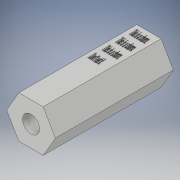
# Autodesk Inventor part: Churro For ARm Gearbox
Saved by Autodesk Inventor 2018 (Build 220112000, 112)
## iProperties
Created: 2019-01-23
Part Number: Churro For ARm Gearbox
Material: Generic
Document SubType Name: Modeling
Designer: Gabriel
Density: 1 g/cm^3
Appearance: Default
Author: Gabriel
Autodesk Inventor part; units mm, degrees
(part 1 of 2)
ref_plane "YZ Plane" through (0, 0, 0) normal (1, 0, 0) x (0, 1, 0)
ref_plane "XZ Plane" through (0, 0, 0) normal (0, 1, 0) x (-1, 0, 0)
ref_plane "XY Plane" through (0, 0, 0) normal (0, 0, 1) x (1, 0, 0)
sketch "Sketch1" plane through (0, 0, 0) normal (0, 0, 1) x (1, 0, 0)
  line L0 (0, 0) -> (0, 6.35) construction
  line L1 (3.6684, 6.35) -> (7.3335, -0.0019)
  line L2 (7.3335, -0.0019) -> (3.6651, -6.3519)
  line L3 (3.6651, -6.3519) -> (-3.6684, -6.35)
  line L4 (-3.6684, -6.35) -> (-7.3335, 0.0019)
  line L5 (-7.3335, 0.0019) -> (-3.6651, 6.3519)
  line L6 (-3.6651, 6.3519) -> (3.6684, 6.35)
  dimension "d0" = 6.35
  constraints: 14 end point, 1 coincident, 1 vertical, 13 other
  measures "d0" distance of L0.start L0.end
extrude "Extrusion1" add sketch "Sketch1" along normal blind 35.56
sketch "Sketch2" plane through (0, 0, 35.56) normal (0, 0, 1) x (1, 0, 0)
  circle A0 centre (0, 0) radius 2.5797
  dimension "d3" = 5.1594
  constraints: 1 centre point, 1 coincident
  measures "d3" diameter of A0
extrude "Extrusion2" cut sketch "Sketch2" against normal blind 38.1
sketch "Sketch3" plane through (-3.6651, 6.3519, 35.56) normal (0.000265, 1, 0) x (1, -0.000265, 0)
  line L0 (1.173, 34.33) -> (52.4364, 34.33) construction
  line L1 (52.4364, 34.33) -> (52.4364, -19.2921) construction
  line L2 (52.4364, -19.2921) -> (1.173, -19.2921) construction
  line L3 (1.173, -19.2921) -> (1.173, 34.33) construction
  line L4 (1.5851, 34.0408) -> (1.4187, 34.0408)
  line L5 (1.4187, 34.0408) -> (1.4187, 31.79)
  line L6 (1.4187, 31.79) -> (1.3533, 31.79)
  line L7 (1.3533, 31.79) -> (1.3533, 34.0408)
  line L8 (1.3533, 34.0408) -> (1.1869, 34.0408)
  line L9 (1.1869, 34.0408) -> (1.1869, 34.33)
  line L10 (1.1869, 34.33) -> (1.5851, 34.33)
  line L11 (1.5851, 34.33) -> (1.5851, 34.0408)
  line L12 (1.9358, 31.79) -> (1.8764, 31.79)
  line L13 (1.8764, 31.79) -> (1.8764, 33.1294)
  spline S0 degree 2 poles (1.8764, 33.1294) (1.8764, 33.2483) (1.8328, 33.4147) (1.8031, 33.4147) knots 0 0 0 1 2 2 2
  spline S1 degree 2 poles (1.8031, 33.4147) (1.7694, 33.4147) (1.706, 33.171) (1.706, 33.0303) knots 0 0 0 1 2 2 2
  line L14 (1.706, 33.0303) -> (1.706, 31.79)
  line L15 (1.706, 31.79) -> (1.6465, 31.79)
  line L16 (1.6465, 31.79) -> (1.6465, 34.33)
  line L17 (1.6465, 34.33) -> (1.706, 34.33)
  line L18 (1.706, 34.33) -> (1.706, 33.4127)
  spline S2 degree 2 poles (1.706, 33.4127) (1.7634, 33.6683) (1.8229, 33.6683) knots 0 0 0 1 1 1
  spline S3 degree 2 poles (1.8229, 33.6683) (1.8684, 33.6683) (1.9358, 33.3929) (1.9358, 33.2086) knots 0 0 0 1 2 2 2
  line L19 (1.9358, 33.2086) -> (1.9358, 31.79)
  line L20 (2.0923, 31.79) -> (2.0329, 31.79)
  line L21 (2.0329, 31.79) -> (2.0329, 33.6188)
  line L22 (2.0329, 33.6188) -> (2.0923, 33.6188)
  line L23 (2.0923, 33.6188) -> (2.0923, 31.79)
  line L24 (2.0923, 33.9675) -> (2.0329, 33.9675)
  line L25 (2.0329, 33.9675) -> (2.0329, 34.33)
  line L26 (2.0329, 34.33) -> (2.0923, 34.33)
  line L27 (2.0923, 34.33) -> (2.0923, 33.9675)
  spline S4 degree 2 poles (2.4609, 32.2913) (2.4609, 32.0238) (2.3776, 31.7128) (2.3142, 31.7128) knots 0 0 0 1 2 2 2
  spline S5 degree 2 poles (2.3142, 31.7128) (2.233, 31.7128) (2.1973, 31.8772) knots 0 0 0 1 1 1
  spline S6 degree 2 poles (2.1973, 31.8772) (2.1676, 32.0159) (2.1656, 32.3289) knots 0 0 0 1 1 1
  line L28 (2.1656, 32.3289) -> (2.2211, 32.3289)
  spline S7 degree 2 poles (2.2211, 32.3289) (2.2211, 32.1447) (2.2508, 32.0436) knots 0 0 0 1 1 1
  spline S8 degree 2 poles (2.2508, 32.0436) (2.2766, 31.9565) (2.3142, 31.9565) knots 0 0 0 1 1 1
  spline S9 degree 2 poles (2.3142, 31.9565) (2.3519, 31.9565) (2.4034, 32.107) (2.4034, 32.2537) knots 0 0 0 1 2 2 2
  spline S10 degree 2 poles (2.4034, 32.2537) (2.4034, 32.4478) (2.3558, 32.5033) knots 0 0 0 1 1 1
  line L29 (2.3558, 32.5033) -> (2.2647, 32.6123)
  spline S11 degree 2 poles (2.2647, 32.6123) (2.2152, 32.6737) (2.1934, 32.8144) knots 0 0 0 1 1 1
  spline S12 degree 2 poles (2.1934, 32.8144) (2.1755, 32.9293) (2.1755, 33.1274) knots 0 0 0 1 1 1
  spline S13 degree 2 poles (2.1755, 33.1274) (2.1755, 33.3751) (2.2528, 33.6703) (2.3162, 33.6703) knots 0 0 0 1 2 2 2
  spline S14 degree 2 poles (2.3162, 33.6703) (2.3776, 33.6703) (2.445, 33.381) (2.447, 33.1056) knots 0 0 0 1 2 2 2
  line L30 (2.447, 33.1056) -> (2.3895, 33.1056)
  spline S15 degree 2 poles (2.3895, 33.1056) (2.3875, 33.3988) (2.3083, 33.3988) knots 0 0 0 1 1 1
  spline S16 degree 2 poles (2.3083, 33.3988) (2.2786, 33.3988) (2.231, 33.2384) (2.231, 33.1175) knots 0 0 0 1 2 2 2
  spline S17 degree 2 poles (2.231, 33.1175) (2.231, 32.9491) (2.2825, 32.8877) knots 0 0 0 1 1 1
  line L31 (2.2825, 32.8877) -> (2.3757, 32.7728)
  spline S18 degree 2 poles (2.3757, 32.7728) (2.4609, 32.6677) (2.4609, 32.2913) knots 0 0 0 1 1 1
  line L32 (2.7897, 31.79) -> (2.7303, 31.79)
  line L33 (2.7303, 31.79) -> (2.7303, 33.6188)
  line L34 (2.7303, 33.6188) -> (2.7897, 33.6188)
  line L35 (2.7897, 33.6188) -> (2.7897, 31.79)
  line L36 (2.7897, 33.9675) -> (2.7303, 33.9675)
  line L37 (2.7303, 33.9675) -> (2.7303, 34.33)
  line L38 (2.7303, 34.33) -> (2.7897, 34.33)
  line L39 (2.7897, 34.33) -> (2.7897, 33.9675)
  spline S19 degree 2 poles (3.1583, 32.2913) (3.1583, 32.0238) (3.075, 31.7128) (3.0116, 31.7128) knots 0 0 0 1 2 2 2
  spline S20 degree 2 poles (3.0116, 31.7128) (2.9304, 31.7128) (2.8948, 31.8772) knots 0 0 0 1 1 1
  spline S21 degree 2 poles (2.8948, 31.8772) (2.865, 32.0159) (2.8631, 32.3289) knots 0 0 0 1 1 1
  line L40 (2.8631, 32.3289) -> (2.9185, 32.3289)
  spline S22 degree 2 poles (2.9185, 32.3289) (2.9185, 32.1447) (2.9482, 32.0436) knots 0 0 0 1 1 1
  spline S23 degree 2 poles (2.9482, 32.0436) (2.974, 31.9565) (3.0116, 31.9565) knots 0 0 0 1 1 1
  spline S24 degree 2 poles (3.0116, 31.9565) (3.0493, 31.9565) (3.1008, 32.107) (3.1008, 32.2537) knots 0 0 0 1 2 2 2
  spline S25 degree 2 poles (3.1008, 32.2537) (3.1008, 32.4478) (3.0533, 32.5033) knots 0 0 0 1 1 1
  line L41 (3.0533, 32.5033) -> (2.9621, 32.6123)
  spline S26 degree 2 poles (2.9621, 32.6123) (2.9126, 32.6737) (2.8908, 32.8144) knots 0 0 0 1 1 1
  spline S27 degree 2 poles (2.8908, 32.8144) (2.873, 32.9293) (2.873, 33.1274) knots 0 0 0 1 1 1
  spline S28 degree 2 poles (2.873, 33.1274) (2.873, 33.3751) (2.9502, 33.6703) (3.0136, 33.6703) knots 0 0 0 1 2 2 2
  spline S29 degree 2 poles (3.0136, 33.6703) (3.075, 33.6703) (3.1424, 33.381) (3.1444, 33.1056) knots 0 0 0 1 2 2 2
  line L42 (3.1444, 33.1056) -> (3.0869, 33.1056)
  spline S30 degree 2 poles (3.0869, 33.1056) (3.085, 33.3988) (3.0057, 33.3988) knots 0 0 0 1 1 1
  spline S31 degree 2 poles (3.0057, 33.3988) (2.976, 33.3988) (2.9284, 33.2384) (2.9284, 33.1175) knots 0 0 0 1 2 2 2
  spline S32 degree 2 poles (2.9284, 33.1175) (2.9284, 32.9491) (2.9799, 32.8877) knots 0 0 0 1 1 1
  line L43 (2.9799, 32.8877) -> (3.0731, 32.7728)
  spline S33 degree 2 poles (3.0731, 32.7728) (3.1583, 32.6677) (3.1583, 32.2913) knots 0 0 0 1 1 1
  spline S34 degree 2 poles (3.7526, 31.7405) (3.7309, 31.7108) (3.7071, 31.7108) knots 0 0 0 1 1 1
  spline S35 degree 2 poles (3.7071, 31.7108) (3.6892, 31.7108) (3.6556, 31.8812) (3.6536, 31.9743) knots 0 0 0 1 2 2 2
  spline S36 degree 2 poles (3.6536, 31.9743) (3.5902, 31.7108) (3.5307, 31.7108) knots 0 0 0 1 1 1
  spline S37 degree 2 poles (3.5307, 31.7108) (3.4753, 31.7108) (3.4099, 31.9961) (3.4099, 32.2477) knots 0 0 0 1 2 2 2
  spline S38 degree 2 poles (3.4099, 32.2477) (3.4099, 32.7212) (3.5228, 32.7985) knots 0 0 0 1 1 1
  line L44 (3.5228, 32.7985) -> (3.6278, 32.8679)
  spline S39 degree 2 poles (3.6278, 32.8679) (3.6516, 32.8857) (3.6516, 33.068) knots 0 0 0 1 1 1
  spline S40 degree 2 poles (3.6516, 33.068) (3.6516, 33.2205) (3.6496, 33.2443) knots 0 0 0 1 1 1
  spline S41 degree 2 poles (3.6496, 33.2443) (3.6437, 33.3176) (3.5902, 33.4087) (3.5565, 33.4087) knots 0 0 0 1 2 2 2
  spline S42 degree 2 poles (3.5565, 33.4087) (3.5228, 33.4087) (3.4872, 33.2522) (3.4812, 33.0719) knots 0 0 0 1 2 2 2
  line L45 (3.4812, 33.0719) -> (3.4277, 33.0719)
  spline S43 degree 2 poles (3.4277, 33.0719) (3.4238, 33.3434) (3.503, 33.6703) (3.5664, 33.6703) knots 0 0 0 1 2 2 2
  spline S44 degree 2 poles (3.5664, 33.6703) (3.6278, 33.6703) (3.713, 33.4543) (3.713, 33.3018) knots 0 0 0 1 2 2 2
  line L46 (3.713, 33.3018) -> (3.713, 32.0654)
  spline S45 degree 2 poles (3.713, 32.0654) (3.713, 32.0278) (3.7269, 31.9664) (3.7368, 31.9584) knots 0 0 0 1 2 2 2
  spline S46 degree 2 poles (3.7368, 31.9584) (3.7427, 31.9545) (3.7526, 31.9584) knots 0 0 0 1 1 1
  line L47 (3.7526, 31.9584) -> (3.7526, 31.7405)
  line L48 (3.6516, 32.3943) -> (3.6516, 32.6777)
  spline S47 degree 2 poles (3.6516, 32.6777) (3.608, 32.6182) (3.5248, 32.5568) knots 0 0 0 1 1 1
  spline S48 degree 2 poles (3.5248, 32.5568) (3.503, 32.535) (3.4713, 32.3606) (3.4713, 32.2517) knots 0 0 0 1 2 2 2
  spline S49 degree 2 poles (3.4713, 32.2517) (3.4713, 32.1269) (3.5089, 31.9584) (3.5367, 31.9584) knots 0 0 0 1 2 2 2
  spline S50 degree 2 poles (3.5367, 31.9584) (3.5842, 31.9584) (3.6516, 32.2239) (3.6516, 32.3943) knots 0 0 0 1 2 2 2
  spline S51 degree 2 poles (4.2935, 32.4201) (4.2856, 32.0377) (4.2381, 31.8554) knots 0 0 0 1 1 1
  spline S52 degree 2 poles (4.2381, 31.8554) (4.2004, 31.7128) (4.143, 31.7128) knots 0 0 0 1 1 1
  spline S53 degree 2 poles (4.143, 31.7128) (4.0697, 31.7128) (3.9825, 32.214) (3.9825, 32.6539) knots 0 0 0 1 2 2 2
  spline S54 degree 2 poles (3.9825, 32.6539) (3.9825, 33.1135) (4.0736, 33.6703) (4.1489, 33.6703) knots 0 0 0 1 2 2 2
  spline S55 degree 2 poles (4.1489, 33.6703) (4.2064, 33.6703) (4.244, 33.5197) knots 0 0 0 1 1 1
  spline S56 degree 2 poles (4.244, 33.5197) (4.2876, 33.3493) (4.2935, 33.0026) knots 0 0 0 1 1 1
  line L49 (4.2935, 33.0026) -> (4.2341, 33.0026)
  spline S57 degree 2 poles (4.2341, 33.0026) (4.2282, 33.3988) (4.1469, 33.3988) knots 0 0 0 1 1 1
  spline S58 degree 2 poles (4.1469, 33.3988) (4.0994, 33.3988) (4.0439, 33.0026) (4.0439, 32.6677) knots 0 0 0 1 2 2 2
  spline S59 degree 2 poles (4.0439, 32.6677) (4.0439, 32.3507) (4.0994, 31.9842) (4.1449, 31.9842) knots 0 0 0 1 2 2 2
  spline S60 degree 2 poles (4.1449, 31.9842) (4.1826, 31.9842) (4.2242, 32.1823) (4.2381, 32.4201) knots 0 0 0 1 2 2 2
  line L50 (4.2381, 32.4201) -> (4.2935, 32.4201)
  line L51 (4.6462, 31.79) -> (4.5868, 31.79)
  line L52 (4.5868, 31.79) -> (4.5868, 33.1294)
  spline S61 degree 2 poles (4.5868, 33.1294) (4.5868, 33.2483) (4.5432, 33.4147) (4.5135, 33.4147) knots 0 0 0 1 2 2 2
  spline S62 degree 2 poles (4.5135, 33.4147) (4.4798, 33.4147) (4.4164, 33.171) (4.4164, 33.0303) knots 0 0 0 1 2 2 2
  line L53 (4.4164, 33.0303) -> (4.4164, 31.79)
  line L54 (4.4164, 31.79) -> (4.3569, 31.79)
  line L55 (4.3569, 31.79) -> (4.3569, 34.33)
  line L56 (4.3569, 34.33) -> (4.4164, 34.33)
  line L57 (4.4164, 34.33) -> (4.4164, 33.4127)
  spline S63 degree 2 poles (4.4164, 33.4127) (4.4738, 33.6683) (4.5333, 33.6683) knots 0 0 0 1 1 1
  spline S64 degree 2 poles (4.5333, 33.6683) (4.5788, 33.6683) (4.6462, 33.3929) (4.6462, 33.2086) knots 0 0 0 1 2 2 2
  line L58 (4.6462, 33.2086) -> (4.6462, 31.79)
  line L59 (5.0345, 31.79) -> (4.9751, 31.79)
  line L60 (4.9751, 31.79) -> (4.9751, 31.9921)
  spline S65 degree 2 poles (4.9751, 31.9921) (4.9533, 31.8376) (4.9295, 31.7782) knots 0 0 0 1 1 1
  spline S66 degree 2 poles (4.9295, 31.7782) (4.9038, 31.7128) (4.8562, 31.7128) knots 0 0 0 1 1 1
  spline S67 degree 2 poles (4.8562, 31.7128) (4.7869, 31.7128) (4.7591, 31.9367) knots 0 0 0 1 1 1
  spline S68 degree 2 poles (4.7591, 31.9367) (4.7433, 32.0575) (4.7433, 32.2081) knots 0 0 0 1 1 1
  line L61 (4.7433, 32.2081) -> (4.7433, 33.6188)
  line L62 (4.7433, 33.6188) -> (4.8027, 33.6188)
  line L63 (4.8027, 33.6188) -> (4.8027, 32.2774)
  spline S69 degree 2 poles (4.8027, 32.2774) (4.8027, 32.1526) (4.8423, 31.9783) (4.8701, 31.9783) knots 0 0 0 1 2 2 2
  spline S70 degree 2 poles (4.8701, 31.9783) (4.9137, 31.9783) (4.9751, 32.2992) (4.9751, 32.5291) knots 0 0 0 1 2 2 2
  line L64 (4.9751, 32.5291) -> (4.9751, 33.6188)
  line L65 (4.9751, 33.6188) -> (5.0345, 33.6188)
  line L66 (5.0345, 33.6188) -> (5.0345, 31.79)
  spline S71 degree 2 poles (5.306, 33.3612) (5.2525, 33.3612) (5.2228, 33.2284) knots 0 0 0 1 1 1
  spline S72 degree 2 poles (5.2228, 33.2284) (5.1891, 33.0818) (5.1891, 32.8144) knots 0 0 0 1 1 1
  line L67 (5.1891, 32.8144) -> (5.1891, 31.79)
  line L68 (5.1891, 31.79) -> (5.1296, 31.79)
  line L69 (5.1296, 31.79) -> (5.1296, 33.6188)
  line L70 (5.1296, 33.6188) -> (5.1891, 33.6188)
  line L71 (5.1891, 33.6188) -> (5.1891, 33.3255)
  spline S73 degree 2 poles (5.1891, 33.3255) (5.2247, 33.6703) (5.2901, 33.6703) knots 0 0 0 1 1 1
  spline S74 degree 2 poles (5.2901, 33.6703) (5.2941, 33.6703) (5.306, 33.6623) knots 0 0 0 1 1 1
  line L72 (5.306, 33.6623) -> (5.306, 33.3612)
  spline S75 degree 2 poles (5.5378, 33.3612) (5.4843, 33.3612) (5.4546, 33.2284) knots 0 0 0 1 1 1
  spline S76 degree 2 poles (5.4546, 33.2284) (5.4209, 33.0818) (5.4209, 32.8144) knots 0 0 0 1 1 1
  line L73 (5.4209, 32.8144) -> (5.4209, 31.79)
  line L74 (5.4209, 31.79) -> (5.3614, 31.79)
  line L75 (5.3614, 31.79) -> (5.3614, 33.6188)
  line L76 (5.3614, 33.6188) -> (5.4209, 33.6188)
  line L77 (5.4209, 33.6188) -> (5.4209, 33.3255)
  spline S77 degree 2 poles (5.4209, 33.3255) (5.4565, 33.6703) (5.5219, 33.6703) knots 0 0 0 1 1 1
  spline S78 degree 2 poles (5.5219, 33.6703) (5.5259, 33.6703) (5.5378, 33.6623) knots 0 0 0 1 1 1
  line L78 (5.5378, 33.6623) -> (5.5378, 33.3612)
  spline S79 degree 2 poles (5.9023, 32.7153) (5.9023, 32.2695) (5.8667, 32.0119) knots 0 0 0 1 1 1
  spline S80 degree 2 poles (5.8667, 32.0119) (5.8231, 31.7128) (5.7379, 31.7128) knots 0 0 0 1 1 1
  spline S81 degree 2 poles (5.7379, 31.7128) (5.6547, 31.7128) (5.6131, 31.9802) knots 0 0 0 1 1 1
  spline S82 degree 2 poles (5.6131, 31.9802) (5.5715, 32.2378) (5.5715, 32.7153) knots 0 0 0 1 1 1
  spline S83 degree 2 poles (5.5715, 32.7153) (5.5715, 33.1611) (5.6567, 33.6703) (5.7379, 33.6703) knots 0 0 0 1 2 2 2
  spline S84 degree 2 poles (5.7379, 33.6703) (5.8171, 33.6703) (5.9023, 33.1611) (5.9023, 32.7153) knots 0 0 0 1 2 2 2
  spline S85 degree 2 poles (5.8409, 32.7153) (5.8409, 33.0264) (5.8092, 33.2106) knots 0 0 0 1 1 1
  spline S86 degree 2 poles (5.8092, 33.2106) (5.7815, 33.377) (5.7379, 33.377) knots 0 0 0 1 1 1
  spline S87 degree 2 poles (5.7379, 33.377) (5.6923, 33.377) (5.6646, 33.2106) knots 0 0 0 1 1 1
  spline S88 degree 2 poles (5.6646, 33.2106) (5.6329, 33.0264) (5.6329, 32.7153) knots 0 0 0 1 1 1
  spline S89 degree 2 poles (5.6329, 32.7153) (5.6329, 32.3923) (5.6903, 32.002) (5.7379, 32.002) knots 0 0 0 1 2 2 2
  spline S90 degree 2 poles (5.7379, 32.002) (5.7835, 32.002) (5.8409, 32.3923) (5.8409, 32.7153) knots 0 0 0 1 2 2 2
  line L79 (6.0648, 31.79) -> (5.9915, 31.79)
  line L80 (5.9915, 31.79) -> (5.9915, 32.1487)
  line L81 (5.9915, 32.1487) -> (6.0648, 32.1487)
  line L82 (6.0648, 32.1487) -> (6.0648, 31.79)
  line L83 (1.5851, 29.9332) -> (1.4187, 29.9332)
  line L84 (1.4187, 29.9332) -> (1.4187, 27.6824)
  line L85 (1.4187, 27.6824) -> (1.3533, 27.6824)
  line L86 (1.3533, 27.6824) -> (1.3533, 29.9332)
  line L87 (1.3533, 29.9332) -> (1.1869, 29.9332)
  line L88 (1.1869, 29.9332) -> (1.1869, 30.2224)
  line L89 (1.1869, 30.2224) -> (1.5851, 30.2224)
  line L90 (1.5851, 30.2224) -> (1.5851, 29.9332)
  line L91 (1.9358, 27.6824) -> (1.8764, 27.6824)
  line L92 (1.8764, 27.6824) -> (1.8764, 29.0218)
  spline S91 degree 2 poles (1.8764, 29.0218) (1.8764, 29.1407) (1.8328, 29.3071) (1.8031, 29.3071) knots 0 0 0 1 2 2 2
  spline S92 degree 2 poles (1.8031, 29.3071) (1.7694, 29.3071) (1.706, 29.0634) (1.706, 28.9227) knots 0 0 0 1 2 2 2
  line L93 (1.706, 28.9227) -> (1.706, 27.6824)
  line L94 (1.706, 27.6824) -> (1.6465, 27.6824)
  line L95 (1.6465, 27.6824) -> (1.6465, 30.2224)
  line L96 (1.6465, 30.2224) -> (1.706, 30.2224)
  line L97 (1.706, 30.2224) -> (1.706, 29.3051)
  spline S93 degree 2 poles (1.706, 29.3051) (1.7634, 29.5607) (1.8229, 29.5607) knots 0 0 0 1 1 1
  spline S94 degree 2 poles (1.8229, 29.5607) (1.8684, 29.5607) (1.9358, 29.2853) (1.9358, 29.101) knots 0 0 0 1 2 2 2
  line L98 (1.9358, 29.101) -> (1.9358, 27.6824)
  line L99 (2.0923, 27.6824) -> (2.0329, 27.6824)
  line L100 (2.0329, 27.6824) -> (2.0329, 29.5112)
  line L101 (2.0329, 29.5112) -> (2.0923, 29.5112)
  line L102 (2.0923, 29.5112) -> (2.0923, 27.6824)
  line L103 (2.0923, 29.8599) -> (2.0329, 29.8599)
  line L104 (2.0329, 29.8599) -> (2.0329, 30.2224)
  line L105 (2.0329, 30.2224) -> (2.0923, 30.2224)
  line L106 (2.0923, 30.2224) -> (2.0923, 29.8599)
  spline S95 degree 2 poles (2.4609, 28.1837) (2.4609, 27.9162) (2.3776, 27.6052) (2.3142, 27.6052) knots 0 0 0 1 2 2 2
  spline S96 degree 2 poles (2.3142, 27.6052) (2.233, 27.6052) (2.1973, 27.7696) knots 0 0 0 1 1 1
  spline S97 degree 2 poles (2.1973, 27.7696) (2.1676, 27.9083) (2.1656, 28.2213) knots 0 0 0 1 1 1
  line L107 (2.1656, 28.2213) -> (2.2211, 28.2213)
  spline S98 degree 2 poles (2.2211, 28.2213) (2.2211, 28.0371) (2.2508, 27.936) knots 0 0 0 1 1 1
  spline S99 degree 2 poles (2.2508, 27.936) (2.2766, 27.8489) (2.3142, 27.8489) knots 0 0 0 1 1 1
  spline S100 degree 2 poles (2.3142, 27.8489) (2.3519, 27.8489) (2.4034, 27.9994) (2.4034, 28.1461) knots 0 0 0 1 2 2 2
  spline S101 degree 2 poles (2.4034, 28.1461) (2.4034, 28.3402) (2.3558, 28.3957) knots 0 0 0 1 1 1
  line L108 (2.3558, 28.3957) -> (2.2647, 28.5047)
  spline S102 degree 2 poles (2.2647, 28.5047) (2.2152, 28.5661) (2.1934, 28.7068) knots 0 0 0 1 1 1
  spline S103 degree 2 poles (2.1934, 28.7068) (2.1755, 28.8217) (2.1755, 29.0198) knots 0 0 0 1 1 1
  spline S104 degree 2 poles (2.1755, 29.0198) (2.1755, 29.2675) (2.2528, 29.5627) (2.3162, 29.5627) knots 0 0 0 1 2 2 2
  spline S105 degree 2 poles (2.3162, 29.5627) (2.3776, 29.5627) (2.445, 29.2734) (2.447, 28.998) knots 0 0 0 1 2 2 2
  line L109 (2.447, 28.998) -> (2.3895, 28.998)
  spline S106 degree 2 poles (2.3895, 28.998) (2.3875, 29.2912) (2.3083, 29.2912) knots 0 0 0 1 1 1
  spline S107 degree 2 poles (2.3083, 29.2912) (2.2786, 29.2912) (2.231, 29.1308) (2.231, 29.0099) knots 0 0 0 1 2 2 2
  spline S108 degree 2 poles (2.231, 29.0099) (2.231, 28.8415) (2.2825, 28.7801) knots 0 0 0 1 1 1
  line L110 (2.2825, 28.7801) -> (2.3757, 28.6652)
  spline S109 degree 2 poles (2.3757, 28.6652) (2.4609, 28.5601) (2.4609, 28.1837) knots 0 0 0 1 1 1
  line L111 (2.7897, 27.6824) -> (2.7303, 27.6824)
  line L112 (2.7303, 27.6824) -> (2.7303, 29.5112)
  line L113 (2.7303, 29.5112) -> (2.7897, 29.5112)
  line L114 (2.7897, 29.5112) -> (2.7897, 27.6824)
  line L115 (2.7897, 29.8599) -> (2.7303, 29.8599)
  line L116 (2.7303, 29.8599) -> (2.7303, 30.2224)
  line L117 (2.7303, 30.2224) -> (2.7897, 30.2224)
  line L118 (2.7897, 30.2224) -> (2.7897, 29.8599)
  spline S110 degree 2 poles (3.1583, 28.1837) (3.1583, 27.9162) (3.075, 27.6052) (3.0116, 27.6052) knots 0 0 0 1 2 2 2
  spline S111 degree 2 poles (3.0116, 27.6052) (2.9304, 27.6052) (2.8948, 27.7696) knots 0 0 0 1 1 1
  spline S112 degree 2 poles (2.8948, 27.7696) (2.865, 27.9083) (2.8631, 28.2213) knots 0 0 0 1 1 1
  line L119 (2.8631, 28.2213) -> (2.9185, 28.2213)
  spline S113 degree 2 poles (2.9185, 28.2213) (2.9185, 28.0371) (2.9482, 27.936) knots 0 0 0 1 1 1
  spline S114 degree 2 poles (2.9482, 27.936) (2.974, 27.8489) (3.0116, 27.8489) knots 0 0 0 1 1 1
  spline S115 degree 2 poles (3.0116, 27.8489) (3.0493, 27.8489) (3.1008, 27.9994) (3.1008, 28.1461) knots 0 0 0 1 2 2 2
  spline S116 degree 2 poles (3.1008, 28.1461) (3.1008, 28.3402) (3.0533, 28.3957) knots 0 0 0 1 1 1
  line L120 (3.0533, 28.3957) -> (2.9621, 28.5047)
  spline S117 degree 2 poles (2.9621, 28.5047) (2.9126, 28.5661) (2.8908, 28.7068) knots 0 0 0 1 1 1
  spline S118 degree 2 poles (2.8908, 28.7068) (2.873, 28.8217) (2.873, 29.0198) knots 0 0 0 1 1 1
  spline S119 degree 2 poles (2.873, 29.0198) (2.873, 29.2675) (2.9502, 29.5627) (3.0136, 29.5627) knots 0 0 0 1 2 2 2
  spline S120 degree 2 poles (3.0136, 29.5627) (3.075, 29.5627) (3.1424, 29.2734) (3.1444, 28.998) knots 0 0 0 1 2 2 2
  line L121 (3.1444, 28.998) -> (3.0869, 28.998)
  spline S121 degree 2 poles (3.0869, 28.998) (3.085, 29.2912) (3.0057, 29.2912) knots 0 0 0 1 1 1
  spline S122 degree 2 poles (3.0057, 29.2912) (2.976, 29.2912) (2.9284, 29.1308) (2.9284, 29.0099) knots 0 0 0 1 2 2 2
  spline S123 degree 2 poles (2.9284, 29.0099) (2.9284, 28.8415) (2.9799, 28.7801) knots 0 0 0 1 1 1
  line L122 (2.9799, 28.7801) -> (3.0731, 28.6652)
  spline S124 degree 2 poles (3.0731, 28.6652) (3.1583, 28.5601) (3.1583, 28.1837) knots 0 0 0 1 1 1
  spline S125 degree 2 poles (3.7526, 27.6329) (3.7309, 27.6032) (3.7071, 27.6032) knots 0 0 0 1 1 1
  spline S126 degree 2 poles (3.7071, 27.6032) (3.6892, 27.6032) (3.6556, 27.7736) (3.6536, 27.8667) knots 0 0 0 1 2 2 2
  spline S127 degree 2 poles (3.6536, 27.8667) (3.5902, 27.6032) (3.5307, 27.6032) knots 0 0 0 1 1 1
  spline S128 degree 2 poles (3.5307, 27.6032) (3.4753, 27.6032) (3.4099, 27.8885) (3.4099, 28.1401) knots 0 0 0 1 2 2 2
  spline S129 degree 2 poles (3.4099, 28.1401) (3.4099, 28.6136) (3.5228, 28.6909) knots 0 0 0 1 1 1
  line L123 (3.5228, 28.6909) -> (3.6278, 28.7603)
  spline S130 degree 2 poles (3.6278, 28.7603) (3.6516, 28.7781) (3.6516, 28.9604) knots 0 0 0 1 1 1
  spline S131 degree 2 poles (3.6516, 28.9604) (3.6516, 29.1129) (3.6496, 29.1367) knots 0 0 0 1 1 1
  spline S132 degree 2 poles (3.6496, 29.1367) (3.6437, 29.21) (3.5902, 29.3011) (3.5565, 29.3011) knots 0 0 0 1 2 2 2
  spline S133 degree 2 poles (3.5565, 29.3011) (3.5228, 29.3011) (3.4872, 29.1446) (3.4812, 28.9643) knots 0 0 0 1 2 2 2
  line L124 (3.4812, 28.9643) -> (3.4277, 28.9643)
  spline S134 degree 2 poles (3.4277, 28.9643) (3.4238, 29.2358) (3.503, 29.5627) (3.5664, 29.5627) knots 0 0 0 1 2 2 2
  spline S135 degree 2 poles (3.5664, 29.5627) (3.6278, 29.5627) (3.713, 29.3467) (3.713, 29.1942) knots 0 0 0 1 2 2 2
  line L125 (3.713, 29.1942) -> (3.713, 27.9578)
  spline S136 degree 2 poles (3.713, 27.9578) (3.713, 27.9202) (3.7269, 27.8588) (3.7368, 27.8508) knots 0 0 0 1 2 2 2
  spline S137 degree 2 poles (3.7368, 27.8508) (3.7427, 27.8469) (3.7526, 27.8508) knots 0 0 0 1 1 1
  line L126 (3.7526, 27.8508) -> (3.7526, 27.6329)
  line L127 (3.6516, 28.2867) -> (3.6516, 28.5701)
  spline S138 degree 2 poles (3.6516, 28.5701) (3.608, 28.5106) (3.5248, 28.4492) knots 0 0 0 1 1 1
  spline S139 degree 2 poles (3.5248, 28.4492) (3.503, 28.4274) (3.4713, 28.253) (3.4713, 28.1441) knots 0 0 0 1 2 2 2
  spline S140 degree 2 poles (3.4713, 28.1441) (3.4713, 28.0193) (3.5089, 27.8508) (3.5367, 27.8508) knots 0 0 0 1 2 2 2
  spline S141 degree 2 poles (3.5367, 27.8508) (3.5842, 27.8508) (3.6516, 28.1163) (3.6516, 28.2867) knots 0 0 0 1 2 2 2
  spline S142 degree 2 poles (4.2935, 28.3125) (4.2856, 27.9301) (4.2381, 27.7478) knots 0 0 0 1 1 1
  spline S143 degree 2 poles (4.2381, 27.7478) (4.2004, 27.6052) (4.143, 27.6052) knots 0 0 0 1 1 1
  spline S144 degree 2 poles (4.143, 27.6052) (4.0697, 27.6052) (3.9825, 28.1064) (3.9825, 28.5463) knots 0 0 0 1 2 2 2
  spline S145 degree 2 poles (3.9825, 28.5463) (3.9825, 29.0059) (4.0736, 29.5627) (4.1489, 29.5627) knots 0 0 0 1 2 2 2
  spline S146 degree 2 poles (4.1489, 29.5627) (4.2064, 29.5627) (4.244, 29.4121) knots 0 0 0 1 1 1
  spline S147 degree 2 poles (4.244, 29.4121) (4.2876, 29.2417) (4.2935, 28.895) knots 0 0 0 1 1 1
  line L128 (4.2935, 28.895) -> (4.2341, 28.895)
  spline S148 degree 2 poles (4.2341, 28.895) (4.2282, 29.2912) (4.1469, 29.2912) knots 0 0 0 1 1 1
  spline S149 degree 2 poles (4.1469, 29.2912) (4.0994, 29.2912) (4.0439, 28.895) (4.0439, 28.5601) knots 0 0 0 1 2 2 2
  spline S150 degree 2 poles (4.0439, 28.5601) (4.0439, 28.2431) (4.0994, 27.8766) (4.1449, 27.8766) knots 0 0 0 1 2 2 2
  spline S151 degree 2 poles (4.1449, 27.8766) (4.1826, 27.8766) (4.2242, 28.0747) (4.2381, 28.3125) knots 0 0 0 1 2 2 2
  line L129 (4.2381, 28.3125) -> (4.2935, 28.3125)
  line L130 (4.6462, 27.6824) -> (4.5868, 27.6824)
  line L131 (4.5868, 27.6824) -> (4.5868, 29.0218)
  spline S152 degree 2 poles (4.5868, 29.0218) (4.5868, 29.1407) (4.5432, 29.3071) (4.5135, 29.3071) knots 0 0 0 1 2 2 2
  spline S153 degree 2 poles (4.5135, 29.3071) (4.4798, 29.3071) (4.4164, 29.0634) (4.4164, 28.9227) knots 0 0 0 1 2 2 2
  line L132 (4.4164, 28.9227) -> (4.4164, 27.6824)
  line L133 (4.4164, 27.6824) -> (4.3569, 27.6824)
  line L134 (4.3569, 27.6824) -> (4.3569, 30.2224)
  line L135 (4.3569, 30.2224) -> (4.4164, 30.2224)
  line L136 (4.4164, 30.2224) -> (4.4164, 29.3051)
  spline S154 degree 2 poles (4.4164, 29.3051) (4.4738, 29.5607) (4.5333, 29.5607) knots 0 0 0 1 1 1
  spline S155 degree 2 poles (4.5333, 29.5607) (4.5788, 29.5607) (4.6462, 29.2853) (4.6462, 29.101) knots 0 0 0 1 2 2 2
  line L137 (4.6462, 29.101) -> (4.6462, 27.6824)
  line L138 (5.0345, 27.6824) -> (4.9751, 27.6824)
  line L139 (4.9751, 27.6824) -> (4.9751, 27.8845)
  spline S156 degree 2 poles (4.9751, 27.8845) (4.9533, 27.73) (4.9295, 27.6706) knots 0 0 0 1 1 1
  spline S157 degree 2 poles (4.9295, 27.6706) (4.9038, 27.6052) (4.8562, 27.6052) knots 0 0 0 1 1 1
  spline S158 degree 2 poles (4.8562, 27.6052) (4.7869, 27.6052) (4.7591, 27.8291) knots 0 0 0 1 1 1
  spline S159 degree 2 poles (4.7591, 27.8291) (4.7433, 27.9499) (4.7433, 28.1005) knots 0 0 0 1 1 1
  line L140 (4.7433, 28.1005) -> (4.7433, 29.5112)
  line L141 (4.7433, 29.5112) -> (4.8027, 29.5112)
  line L142 (4.8027, 29.5112) -> (4.8027, 28.1698)
  spline S160 degree 2 poles (4.8027, 28.1698) (4.8027, 28.045) (4.8423, 27.8707) (4.8701, 27.8707) knots 0 0 0 1 2 2 2
  spline S161 degree 2 poles (4.8701, 27.8707) (4.9137, 27.8707) (4.9751, 28.1916) (4.9751, 28.4215) knots 0 0 0 1 2 2 2
  line L143 (4.9751, 28.4215) -> (4.9751, 29.5112)
  line L144 (4.9751, 29.5112) -> (5.0345, 29.5112)
  line L145 (5.0345, 29.5112) -> (5.0345, 27.6824)
  spline S162 degree 2 poles (5.306, 29.2536) (5.2525, 29.2536) (5.2228, 29.1208) knots 0 0 0 1 1 1
  spline S163 degree 2 poles (5.2228, 29.1208) (5.1891, 28.9742) (5.1891, 28.7068) knots 0 0 0 1 1 1
  line L146 (5.1891, 28.7068) -> (5.1891, 27.6824)
  line L147 (5.1891, 27.6824) -> (5.1296, 27.6824)
  line L148 (5.1296, 27.6824) -> (5.1296, 29.5112)
  line L149 (5.1296, 29.5112) -> (5.1891, 29.5112)
  line L150 (5.1891, 29.5112) -> (5.1891, 29.2179)
  spline S164 degree 2 poles (5.1891, 29.2179) (5.2247, 29.5627) (5.2901, 29.5627) knots 0 0 0 1 1 1
  spline S165 degree 2 poles (5.2901, 29.5627) (5.2941, 29.5627) (5.306, 29.5547) knots 0 0 0 1 1 1
  line L151 (5.306, 29.5547) -> (5.306, 29.2536)
  spline S166 degree 2 poles (5.5378, 29.2536) (5.4843, 29.2536) (5.4546, 29.1208) knots 0 0 0 1 1 1
  spline S167 degree 2 poles (5.4546, 29.1208) (5.4209, 28.9742) (5.4209, 28.7068) knots 0 0 0 1 1 1
  line L152 (5.4209, 28.7068) -> (5.4209, 27.6824)
  line L153 (5.4209, 27.6824) -> (5.3614, 27.6824)
  line L154 (5.3614, 27.6824) -> (5.3614, 29.5112)
  line L155 (5.3614, 29.5112) -> (5.4209, 29.5112)
  line L156 (5.4209, 29.5112) -> (5.4209, 29.2179)
  spline S168 degree 2 poles (5.4209, 29.2179) (5.4565, 29.5627) (5.5219, 29.5627) knots 0 0 0 1 1 1
  spline S169 degree 2 poles (5.5219, 29.5627) (5.5259, 29.5627) (5.5378, 29.5547) knots 0 0 0 1 1 1
  line L157 (5.5378, 29.5547) -> (5.5378, 29.2536)
  spline S170 degree 2 poles (5.9023, 28.6077) (5.9023, 28.1619) (5.8667, 27.9043) knots 0 0 0 1 1 1
  spline S171 degree 2 poles (5.8667, 27.9043) (5.8231, 27.6052) (5.7379, 27.6052) knots 0 0 0 1 1 1
  spline S172 degree 2 poles (5.7379, 27.6052) (5.6547, 27.6052) (5.6131, 27.8726) knots 0 0 0 1 1 1
  spline S173 degree 2 poles (5.6131, 27.8726) (5.5715, 28.1302) (5.5715, 28.6077) knots 0 0 0 1 1 1
  spline S174 degree 2 poles (5.5715, 28.6077) (5.5715, 29.0535) (5.6567, 29.5627) (5.7379, 29.5627) knots 0 0 0 1 2 2 2
  spline S175 degree 2 poles (5.7379, 29.5627) (5.8171, 29.5627) (5.9023, 29.0535) (5.9023, 28.6077) knots 0 0 0 1 2 2 2
  spline S176 degree 2 poles (5.8409, 28.6077) (5.8409, 28.9188) (5.8092, 29.103) knots 0 0 0 1 1 1
  spline S177 degree 2 poles (5.8092, 29.103) (5.7815, 29.2694) (5.7379, 29.2694) knots 0 0 0 1 1 1
  spline S178 degree 2 poles (5.7379, 29.2694) (5.6923, 29.2694) (5.6646, 29.103) knots 0 0 0 1 1 1
  spline S179 degree 2 poles (5.6646, 29.103) (5.6329, 28.9188) (5.6329, 28.6077) knots 0 0 0 1 1 1
  spline S180 degree 2 poles (5.6329, 28.6077) (5.6329, 28.2847) (5.6903, 27.8944) (5.7379, 27.8944) knots 0 0 0 1 2 2 2
  spline S181 degree 2 poles (5.7379, 27.8944) (5.7835, 27.8944) (5.8409, 28.2847) (5.8409, 28.6077) knots 0 0 0 1 2 2 2
  line L158 (6.0648, 27.6824) -> (5.9915, 27.6824)
  line L159 (5.9915, 27.6824) -> (5.9915, 28.0411)
  line L160 (5.9915, 28.0411) -> (6.0648, 28.0411)
  line L161 (6.0648, 28.0411) -> (6.0648, 27.6824)
  line L162 (1.5851, 25.8256) -> (1.4187, 25.8256)
  line L163 (1.4187, 25.8256) -> (1.4187, 23.5748)
  line L164 (1.4187, 23.5748) -> (1.3533, 23.5748)
  line L165 (1.3533, 23.5748) -> (1.3533, 25.8256)
  line L166 (1.3533, 25.8256) -> (1.1869, 25.8256)
  line L167 (1.1869, 25.8256) -> (1.1869, 26.1148)
  line L168 (1.1869, 26.1148) -> (1.5851, 26.1148)
  line L169 (1.5851, 26.1148) -> (1.5851, 25.8256)
  line L170 (1.9358, 23.5748) -> (1.8764, 23.5748)
  line L171 (1.8764, 23.5748) -> (1.8764, 24.9142)
  spline S182 degree 2 poles (1.8764, 24.9142) (1.8764, 25.0331) (1.8328, 25.1995) (1.8031, 25.1995) knots 0 0 0 1 2 2 2
  spline S183 degree 2 poles (1.8031, 25.1995) (1.7694, 25.1995) (1.706, 24.9558) (1.706, 24.8151) knots 0 0 0 1 2 2 2
  line L172 (1.706, 24.8151) -> (1.706, 23.5748)
  line L173 (1.706, 23.5748) -> (1.6465, 23.5748)
  line L174 (1.6465, 23.5748) -> (1.6465, 26.1148)
  line L175 (1.6465, 26.1148) -> (1.706, 26.1148)
  line L176 (1.706, 26.1148) -> (1.706, 25.1975)
  spline S184 degree 2 poles (1.706, 25.1975) (1.7634, 25.4531) (1.8229, 25.4531) knots 0 0 0 1 1 1
  spline S185 degree 2 poles (1.8229, 25.4531) (1.8684, 25.4531) (1.9358, 25.1777) (1.9358, 24.9934) knots 0 0 0 1 2 2 2
  line L177 (1.9358, 24.9934) -> (1.9358, 23.5748)
  line L178 (2.0923, 23.5748) -> (2.0329, 23.5748)
  line L179 (2.0329, 23.5748) -> (2.0329, 25.4036)
  line L180 (2.0329, 25.4036) -> (2.0923, 25.4036)
  line L181 (2.0923, 25.4036) -> (2.0923, 23.5748)
  line L182 (2.0923, 25.7523) -> (2.0329, 25.7523)
  line L183 (2.0329, 25.7523) -> (2.0329, 26.1148)
  line L184 (2.0329, 26.1148) -> (2.0923, 26.1148)
  line L185 (2.0923, 26.1148) -> (2.0923, 25.7523)
  spline S186 degree 2 poles (2.4609, 24.0761) (2.4609, 23.8086) (2.3776, 23.4976) (2.3142, 23.4976) knots 0 0 0 1 2 2 2
  spline S187 degree 2 poles (2.3142, 23.4976) (2.233, 23.4976) (2.1973, 23.662) knots 0 0 0 1 1 1
  spline S188 degree 2 poles (2.1973, 23.662) (2.1676, 23.8007) (2.1656, 24.1137) knots 0 0 0 1 1 1
  line L186 (2.1656, 24.1137) -> (2.2211, 24.1137)
  spline S189 degree 2 poles (2.2211, 24.1137) (2.2211, 23.9295) (2.2508, 23.8284) knots 0 0 0 1 1 1
  spline S190 degree 2 poles (2.2508, 23.8284) (2.2766, 23.7413) (2.3142, 23.7413) knots 0 0 0 1 1 1
  spline S191 degree 2 poles (2.3142, 23.7413) (2.3519, 23.7413) (2.4034, 23.8918) (2.4034, 24.0385) knots 0 0 0 1 2 2 2
  spline S192 degree 2 poles (2.4034, 24.0385) (2.4034, 24.2326) (2.3558, 24.2881) knots 0 0 0 1 1 1
  line L187 (2.3558, 24.2881) -> (2.2647, 24.3971)
  spline S193 degree 2 poles (2.2647, 24.3971) (2.2152, 24.4585) (2.1934, 24.5992) knots 0 0 0 1 1 1
  spline S194 degree 2 poles (2.1934, 24.5992) (2.1755, 24.7141) (2.1755, 24.9122) knots 0 0 0 1 1 1
  spline S195 degree 2 poles (2.1755, 24.9122) (2.1755, 25.1599) (2.2528, 25.4551) (2.3162, 25.4551) knots 0 0 0 1 2 2 2
  spline S196 degree 2 poles (2.3162, 25.4551) (2.3776, 25.4551) (2.445, 25.1658) (2.447, 24.8904) knots 0 0 0 1 2 2 2
  line L188 (2.447, 24.8904) -> (2.3895, 24.8904)
  spline S197 degree 2 poles (2.3895, 24.8904) (2.3875, 25.1836) (2.3083, 25.1836) knots 0 0 0 1 1 1
  spline S198 degree 2 poles (2.3083, 25.1836) (2.2786, 25.1836) (2.231, 25.0232) (2.231, 24.9023) knots 0 0 0 1 2 2 2
  spline S199 degree 2 poles (2.231, 24.9023) (2.231, 24.7339) (2.2825, 24.6725) knots 0 0 0 1 1 1
  line L189 (2.2825, 24.6725) -> (2.3757, 24.5576)
  spline S200 degree 2 poles (2.3757, 24.5576) (2.4609, 24.4525) (2.4609, 24.0761) knots 0 0 0 1 1 1
  line L190 (2.7897, 23.5748) -> (2.7303, 23.5748)
  line L191 (2.7303, 23.5748) -> (2.7303, 25.4036)
  line L192 (2.7303, 25.4036) -> (2.7897, 25.4036)
  line L193 (2.7897, 25.4036) -> (2.7897, 23.5748)
  line L194 (2.7897, 25.7523) -> (2.7303, 25.7523)
  line L195 (2.7303, 25.7523) -> (2.7303, 26.1148)
  line L196 (2.7303, 26.1148) -> (2.7897, 26.1148)
  line L197 (2.7897, 26.1148) -> (2.7897, 25.7523)
  spline S201 degree 2 poles (3.1583, 24.0761) (3.1583, 23.8086) (3.075, 23.4976) (3.0116, 23.4976) knots 0 0 0 1 2 2 2
  spline S202 degree 2 poles (3.0116, 23.4976) (2.9304, 23.4976) (2.8948, 23.662) knots 0 0 0 1 1 1
  spline S203 degree 2 poles (2.8948, 23.662) (2.865, 23.8007) (2.8631, 24.1137) knots 0 0 0 1 1 1
  line L198 (2.8631, 24.1137) -> (2.9185, 24.1137)
  spline S204 degree 2 poles (2.9185, 24.1137) (2.9185, 23.9295) (2.9482, 23.8284) knots 0 0 0 1 1 1
  spline S205 degree 2 poles (2.9482, 23.8284) (2.974, 23.7413) (3.0116, 23.7413) knots 0 0 0 1 1 1
  spline S206 degree 2 poles (3.0116, 23.7413) (3.0493, 23.7413) (3.1008, 23.8918) (3.1008, 24.0385) knots 0 0 0 1 2 2 2
  spline S207 degree 2 poles (3.1008, 24.0385) (3.1008, 24.2326) (3.0533, 24.2881) knots 0 0 0 1 1 1
  line L199 (3.0533, 24.2881) -> (2.9621, 24.3971)
  spline S208 degree 2 poles (2.9621, 24.3971) (2.9126, 24.4585) (2.8908, 24.5992) knots 0 0 0 1 1 1
  spline S209 degree 2 poles (2.8908, 24.5992) (2.873, 24.7141) (2.873, 24.9122) knots 0 0 0 1 1 1
  spline S210 degree 2 poles (2.873, 24.9122) (2.873, 25.1599) (2.9502, 25.4551) (3.0136, 25.4551) knots 0 0 0 1 2 2 2
  spline S211 degree 2 poles (3.0136, 25.4551) (3.075, 25.4551) (3.1424, 25.1658) (3.1444, 24.8904) knots 0 0 0 1 2 2 2
  line L200 (3.1444, 24.8904) -> (3.0869, 24.8904)
  spline S212 degree 2 poles (3.0869, 24.8904) (3.085, 25.1836) (3.0057, 25.1836) knots 0 0 0 1 1 1
  spline S213 degree 2 poles (3.0057, 25.1836) (2.976, 25.1836) (2.9284, 25.0232) (2.9284, 24.9023) knots 0 0 0 1 2 2 2
  spline S214 degree 2 poles (2.9284, 24.9023) (2.9284, 24.7339) (2.9799, 24.6725) knots 0 0 0 1 1 1
  line L201 (2.9799, 24.6725) -> (3.0731, 24.5576)
  spline S215 degree 2 poles (3.0731, 24.5576) (3.1583, 24.4525) (3.1583, 24.0761) knots 0 0 0 1 1 1
  spline S216 degree 2 poles (3.7526, 23.5253) (3.7309, 23.4956) (3.7071, 23.4956) knots 0 0 0 1 1 1
  spline S217 degree 2 poles (3.7071, 23.4956) (3.6892, 23.4956) (3.6556, 23.666) (3.6536, 23.7591) knots 0 0 0 1 2 2 2
  spline S218 degree 2 poles (3.6536, 23.7591) (3.5902, 23.4956) (3.5307, 23.4956) knots 0 0 0 1 1 1
  spline S219 degree 2 poles (3.5307, 23.4956) (3.4753, 23.4956) (3.4099, 23.7809) (3.4099, 24.0325) knots 0 0 0 1 2 2 2
  spline S220 degree 2 poles (3.4099, 24.0325) (3.4099, 24.506) (3.5228, 24.5833) knots 0 0 0 1 1 1
  line L202 (3.5228, 24.5833) -> (3.6278, 24.6527)
  spline S221 degree 2 poles (3.6278, 24.6527) (3.6516, 24.6705) (3.6516, 24.8528) knots 0 0 0 1 1 1
  spline S222 degree 2 poles (3.6516, 24.8528) (3.6516, 25.0053) (3.6496, 25.0291) knots 0 0 0 1 1 1
  spline S223 degree 2 poles (3.6496, 25.0291) (3.6437, 25.1024) (3.5902, 25.1935) (3.5565, 25.1935) knots 0 0 0 1 2 2 2
  spline S224 degree 2 poles (3.5565, 25.1935) (3.5228, 25.1935) (3.4872, 25.037) (3.4812, 24.8567) knots 0 0 0 1 2 2 2
  line L203 (3.4812, 24.8567) -> (3.4277, 24.8567)
  spline S225 degree 2 poles (3.4277, 24.8567) (3.4238, 25.1282) (3.503, 25.4551) (3.5664, 25.4551) knots 0 0 0 1 2 2 2
  spline S226 degree 2 poles (3.5664, 25.4551) (3.6278, 25.4551) (3.713, 25.2391) (3.713, 25.0866) knots 0 0 0 1 2 2 2
  line L204 (3.713, 25.0866) -> (3.713, 23.8502)
  spline S227 degree 2 poles (3.713, 23.8502) (3.713, 23.8126) (3.7269, 23.7512) (3.7368, 23.7432) knots 0 0 0 1 2 2 2
  spline S228 degree 2 poles (3.7368, 23.7432) (3.7427, 23.7393) (3.7526, 23.7432) knots 0 0 0 1 1 1
  line L205 (3.7526, 23.7432) -> (3.7526, 23.5253)
  line L206 (3.6516, 24.1791) -> (3.6516, 24.4625)
  spline S229 degree 2 poles (3.6516, 24.4625) (3.608, 24.403) (3.5248, 24.3416) knots 0 0 0 1 1 1
  spline S230 degree 2 poles (3.5248, 24.3416) (3.503, 24.3198) (3.4713, 24.1454) (3.4713, 24.0365) knots 0 0 0 1 2 2 2
  spline S231 degree 2 poles (3.4713, 24.0365) (3.4713, 23.9117) (3.5089, 23.7432) (3.5367, 23.7432) knots 0 0 0 1 2 2 2
  spline S232 degree 2 poles (3.5367, 23.7432) (3.5842, 23.7432) (3.6516, 24.0087) (3.6516, 24.1791) knots 0 0 0 1 2 2 2
  spline S233 degree 2 poles (4.2935, 24.2049) (4.2856, 23.8225) (4.2381, 23.6402) knots 0 0 0 1 1 1
  spline S234 degree 2 poles (4.2381, 23.6402) (4.2004, 23.4976) (4.143, 23.4976) knots 0 0 0 1 1 1
  spline S235 degree 2 poles (4.143, 23.4976) (4.0697, 23.4976) (3.9825, 23.9988) (3.9825, 24.4387) knots 0 0 0 1 2 2 2
  spline S236 degree 2 poles (3.9825, 24.4387) (3.9825, 24.8983) (4.0736, 25.4551) (4.1489, 25.4551) knots 0 0 0 1 2 2 2
  spline S237 degree 2 poles (4.1489, 25.4551) (4.2064, 25.4551) (4.244, 25.3045) knots 0 0 0 1 1 1
  spline S238 degree 2 poles (4.244, 25.3045) (4.2876, 25.1341) (4.2935, 24.7874) knots 0 0 0 1 1 1
  line L207 (4.2935, 24.7874) -> (4.2341, 24.7874)
  spline S239 degree 2 poles (4.2341, 24.7874) (4.2282, 25.1836) (4.1469, 25.1836) knots 0 0 0 1 1 1
  spline S240 degree 2 poles (4.1469, 25.1836) (4.0994, 25.1836) (4.0439, 24.7874) (4.0439, 24.4525) knots 0 0 0 1 2 2 2
  spline S241 degree 2 poles (4.0439, 24.4525) (4.0439, 24.1355) (4.0994, 23.769) (4.1449, 23.769) knots 0 0 0 1 2 2 2
  spline S242 degree 2 poles (4.1449, 23.769) (4.1826, 23.769) (4.2242, 23.9671) (4.2381, 24.2049) knots 0 0 0 1 2 2 2
  line L208 (4.2381, 24.2049) -> (4.2935, 24.2049)
  line L209 (4.6462, 23.5748) -> (4.5868, 23.5748)
  line L210 (4.5868, 23.5748) -> (4.5868, 24.9142)
  spline S243 degree 2 poles (4.5868, 24.9142) (4.5868, 25.0331) (4.5432, 25.1995) (4.5135, 25.1995) knots 0 0 0 1 2 2 2
  spline S244 degree 2 poles (4.5135, 25.1995) (4.4798, 25.1995) (4.4164, 24.9558) (4.4164, 24.8151) knots 0 0 0 1 2 2 2
  line L211 (4.4164, 24.8151) -> (4.4164, 23.5748)
  line L212 (4.4164, 23.5748) -> (4.3569, 23.5748)
  line L213 (4.3569, 23.5748) -> (4.3569, 26.1148)
  line L214 (4.3569, 26.1148) -> (4.4164, 26.1148)
  line L215 (4.4164, 26.1148) -> (4.4164, 25.1975)
  spline S245 degree 2 poles (4.4164, 25.1975) (4.4738, 25.4531) (4.5333, 25.4531) knots 0 0 0 1 1 1
  spline S246 degree 2 poles (4.5333, 25.4531) (4.5788, 25.4531) (4.6462, 25.1777) (4.6462, 24.9934) knots 0 0 0 1 2 2 2
  line L216 (4.6462, 24.9934) -> (4.6462, 23.5748)
  line L217 (5.0345, 23.5748) -> (4.9751, 23.5748)
  line L218 (4.9751, 23.5748) -> (4.9751, 23.7769)
  spline S247 degree 2 poles (4.9751, 23.7769) (4.9533, 23.6224) (4.9295, 23.563) knots 0 0 0 1 1 1
  spline S248 degree 2 poles (4.9295, 23.563) (4.9038, 23.4976) (4.8562, 23.4976) knots 0 0 0 1 1 1
  spline S249 degree 2 poles (4.8562, 23.4976) (4.7869, 23.4976) (4.7591, 23.7215) knots 0 0 0 1 1 1
  spline S250 degree 2 poles (4.7591, 23.7215) (4.7433, 23.8423) (4.7433, 23.9929) knots 0 0 0 1 1 1
  line L219 (4.7433, 23.9929) -> (4.7433, 25.4036)
  line L220 (4.7433, 25.4036) -> (4.8027, 25.4036)
  line L221 (4.8027, 25.4036) -> (4.8027, 24.0622)
  spline S251 degree 2 poles (4.8027, 24.0622) (4.8027, 23.9374) (4.8423, 23.7631) (4.8701, 23.7631) knots 0 0 0 1 2 2 2
  spline S252 degree 2 poles (4.8701, 23.7631) (4.9137, 23.7631) (4.9751, 24.084) (4.9751, 24.3139) knots 0 0 0 1 2 2 2
  line L222 (4.9751, 24.3139) -> (4.9751, 25.4036)
  line L223 (4.9751, 25.4036) -> (5.0345, 25.4036)
  line L224 (5.0345, 25.4036) -> (5.0345, 23.5748)
  spline S253 degree 2 poles (5.306, 25.146) (5.2525, 25.146) (5.2228, 25.0132) knots 0 0 0 1 1 1
  spline S254 degree 2 poles (5.2228, 25.0132) (5.1891, 24.8666) (5.1891, 24.5992) knots 0 0 0 1 1 1
  line L225 (5.1891, 24.5992) -> (5.1891, 23.5748)
  line L226 (5.1891, 23.5748) -> (5.1296, 23.5748)
  line L227 (5.1296, 23.5748) -> (5.1296, 25.4036)
  line L228 (5.1296, 25.4036) -> (5.1891, 25.4036)
  line L229 (5.1891, 25.4036) -> (5.1891, 25.1103)
  spline S255 degree 2 poles (5.1891, 25.1103) (5.2247, 25.4551) (5.2901, 25.4551) knots 0 0 0 1 1 1
  spline S256 degree 2 poles (5.2901, 25.4551) (5.2941, 25.4551) (5.306, 25.4471) knots 0 0 0 1 1 1
  line L230 (5.306, 25.4471) -> (5.306, 25.146)
  spline S257 degree 2 poles (5.5378, 25.146) (5.4843, 25.146) (5.4546, 25.0132) knots 0 0 0 1 1 1
  spline S258 degree 2 poles (5.4546, 25.0132) (5.4209, 24.8666) (5.4209, 24.5992) knots 0 0 0 1 1 1
  line L231 (5.4209, 24.5992) -> (5.4209, 23.5748)
  line L232 (5.4209, 23.5748) -> (5.3614, 23.5748)
  line L233 (5.3614, 23.5748) -> (5.3614, 25.4036)
  line L234 (5.3614, 25.4036) -> (5.4209, 25.4036)
  line L235 (5.4209, 25.4036) -> (5.4209, 25.1103)
  spline S259 degree 2 poles (5.4209, 25.1103) (5.4565, 25.4551) (5.5219, 25.4551) knots 0 0 0 1 1 1
  spline S260 degree 2 poles (5.5219, 25.4551) (5.5259, 25.4551) (5.5378, 25.4471) knots 0 0 0 1 1 1
  line L236 (5.5378, 25.4471) -> (5.5378, 25.146)
  spline S261 degree 2 poles (5.9023, 24.5001) (5.9023, 24.0543) (5.8667, 23.7967) knots 0 0 0 1 1 1
  spline S262 degree 2 poles (5.8667, 23.7967) (5.8231, 23.4976) (5.7379, 23.4976) knots 0 0 0 1 1 1
  spline S263 degree 2 poles (5.7379, 23.4976) (5.6547, 23.4976) (5.6131, 23.765) knots 0 0 0 1 1 1
  spline S264 degree 2 poles (5.6131, 23.765) (5.5715, 24.0226) (5.5715, 24.5001) knots 0 0 0 1 1 1
  spline S265 degree 2 poles (5.5715, 24.5001) (5.5715, 24.9459) (5.6567, 25.4551) (5.7379, 25.4551) knots 0 0 0 1 2 2 2
  spline S266 degree 2 poles (5.7379, 25.4551) (5.8171, 25.4551) (5.9023, 24.9459) (5.9023, 24.5001) knots 0 0 0 1 2 2 2
  spline S267 degree 2 poles (5.8409, 24.5001) (5.8409, 24.8112) (5.8092, 24.9954) knots 0 0 0 1 1 1
  spline S268 degree 2 poles (5.8092, 24.9954) (5.7815, 25.1618) (5.7379, 25.1618) knots 0 0 0 1 1 1
  spline S269 degree 2 poles (5.7379, 25.1618) (5.6923, 25.1618) (5.6646, 24.9954) knots 0 0 0 1 1 1
  spline S270 degree 2 poles (5.6646, 24.9954) (5.6329, 24.8112) (5.6329, 24.5001) knots 0 0 0 1 1 1
  spline S271 degree 2 poles (5.6329, 24.5001) (5.6329, 24.1771) (5.6903, 23.7868) (5.7379, 23.7868) knots 0 0 0 1 2 2 2
  spline S272 degree 2 poles (5.7379, 23.7868) (5.7835, 23.7868) (5.8409, 24.1771) (5.8409, 24.5001) knots 0 0 0 1 2 2 2
  line L237 (6.0648, 23.5748) -> (5.9915, 23.5748)
  line L238 (5.9915, 23.5748) -> (5.9915, 23.9334)
  line L239 (5.9915, 23.9334) -> (6.0648, 23.9334)
  line L240 (6.0648, 23.9334) -> (6.0648, 23.5748)
  spline S273 degree 2 poles (1.6366, 20.759) (1.6366, 20.1825) (1.5752, 19.8021) knots 0 0 0 1 1 1
  spline S274 degree 2 poles (1.5752, 19.8021) (1.5217, 19.4672) (1.4563, 19.4672) knots 0 0 0 1 1 1
  line L241 (1.4563, 19.4672) -> (1.2344, 19.4672)
  line L242 (1.2344, 19.4672) -> (1.2344, 22.0072)
  line L243 (1.2344, 22.0072) -> (1.4405, 22.0072)
  spline S275 degree 2 poles (1.4405, 22.0072) (1.5118, 22.0072) (1.5673, 21.7279) knots 0 0 0 1 1 1
  spline S276 degree 2 poles (1.5673, 21.7279) (1.6366, 21.3831) (1.6366, 20.759) knots 0 0 0 1 1 1
  spline S277 degree 2 poles (1.5713, 20.759) (1.5713, 21.2227) (1.5316, 21.4782) knots 0 0 0 1 1 1
  spline S278 degree 2 poles (1.5316, 21.4782) (1.494, 21.718) (1.4306, 21.718) knots 0 0 0 1 1 1
  line L244 (1.4306, 21.718) -> (1.2998, 21.718)
  line L245 (1.2998, 21.718) -> (1.2998, 19.7565)
  line L246 (1.2998, 19.7565) -> (1.4464, 19.7565)
  spline S279 degree 2 poles (1.4464, 19.7565) (1.5059, 19.7565) (1.5396, 20.0378) knots 0 0 0 1 1 1
  spline S280 degree 2 poles (1.5396, 20.0378) (1.5713, 20.3113) (1.5713, 20.759) knots 0 0 0 1 1 1
  spline S281 degree 2 poles (2.0329, 20.3925) (2.0329, 19.9467) (1.9972, 19.6891) knots 0 0 0 1 1 1
  spline S282 degree 2 poles (1.9972, 19.6891) (1.9536, 19.39) (1.8684, 19.39) knots 0 0 0 1 1 1
  spline S283 degree 2 poles (1.8684, 19.39) (1.7852, 19.39) (1.7436, 19.6574) knots 0 0 0 1 1 1
  spline S284 degree 2 poles (1.7436, 19.6574) (1.702, 19.915) (1.702, 20.3925) knots 0 0 0 1 1 1
  spline S285 degree 2 poles (1.702, 20.3925) (1.702, 20.8383) (1.7872, 21.3475) (1.8684, 21.3475) knots 0 0 0 1 2 2 2
  spline S286 degree 2 poles (1.8684, 21.3475) (1.9477, 21.3475) (2.0329, 20.8383) (2.0329, 20.3925) knots 0 0 0 1 2 2 2
  spline S287 degree 2 poles (1.9715, 20.3925) (1.9715, 20.7036) (1.9398, 20.8878) knots 0 0 0 1 1 1
  spline S288 degree 2 poles (1.9398, 20.8878) (1.912, 21.0542) (1.8684, 21.0542) knots 0 0 0 1 1 1
  spline S289 degree 2 poles (1.8684, 21.0542) (1.8229, 21.0542) (1.7951, 20.8878) knots 0 0 0 1 1 1
  spline S290 degree 2 poles (1.7951, 20.8878) (1.7634, 20.7036) (1.7634, 20.3925) knots 0 0 0 1 1 1
  spline S291 degree 2 poles (1.7634, 20.3925) (1.7634, 20.0695) (1.8209, 19.6792) (1.8684, 19.6792) knots 0 0 0 1 2 2 2
  spline S292 degree 2 poles (1.8684, 19.6792) (1.914, 19.6792) (1.9715, 20.0695) (1.9715, 20.3925) knots 0 0 0 1 2 2 2
  line L247 (2.4014, 19.4672) -> (2.342, 19.4672)
  line L248 (2.342, 19.4672) -> (2.342, 20.7967)
  spline S293 degree 2 poles (2.342, 20.7967) (2.342, 20.9037) (2.2984, 21.082) (2.2687, 21.082) knots 0 0 0 1 2 2 2
  spline S294 degree 2 poles (2.2687, 21.082) (2.2251, 21.082) (2.1696, 20.765) (2.1696, 20.5213) knots 0 0 0 1 2 2 2
  line L249 (2.1696, 20.5213) -> (2.1696, 19.4672)
  line L250 (2.1696, 19.4672) -> (2.1102, 19.4672)
  line L251 (2.1102, 19.4672) -> (2.1102, 21.296)
  line L252 (2.1102, 21.296) -> (2.1696, 21.296)
  line L253 (2.1696, 21.296) -> (2.1696, 21.0582)
  spline S295 degree 2 poles (2.1696, 21.0582) (2.2072, 21.3475) (2.2766, 21.3475) knots 0 0 0 1 1 1
  spline S296 degree 2 poles (2.2766, 21.3475) (2.344, 21.3475) (2.3757, 21.1771) knots 0 0 0 1 1 1
  spline S297 degree 2 poles (2.3757, 21.1771) (2.4014, 21.0443) (2.4014, 20.8422) knots 0 0 0 1 1 1
  line L254 (2.4014, 20.8422) -> (2.4014, 19.4672)
  line L255 (2.548, 21.5357) -> (2.5302, 21.076)
  line L256 (2.5302, 21.076) -> (2.5025, 21.076)
  line L257 (2.5025, 21.076) -> (2.4826, 21.5436)
  line L258 (2.4826, 21.5436) -> (2.4826, 21.9339)
  line L259 (2.4826, 21.9339) -> (2.548, 21.9339)
  line L260 (2.548, 21.9339) -> (2.548, 21.5357)
  spline S298 degree 2 poles (2.76, 19.4078) (2.7343, 19.384) (2.7105, 19.384) knots 0 0 0 1 1 1
  spline S299 degree 2 poles (2.7105, 19.384) (2.6808, 19.384) (2.661, 19.4712) knots 0 0 0 1 1 1
  spline S300 degree 2 poles (2.661, 19.4712) (2.6451, 19.5485) (2.6451, 19.6495) knots 0 0 0 1 1 1
  line L261 (2.6451, 19.6495) -> (2.6451, 21.0285)
  line L262 (2.6451, 21.0285) -> (2.5936, 21.0285)
  line L263 (2.5936, 21.0285) -> (2.5936, 21.296)
  line L264 (2.5936, 21.296) -> (2.6451, 21.296)
  line L265 (2.6451, 21.296) -> (2.6451, 21.7913)
  line L266 (2.6451, 21.7913) -> (2.7045, 21.7913)
  line L267 (2.7045, 21.7913) -> (2.7045, 21.296)
  line L268 (2.7045, 21.296) -> (2.76, 21.296)
  line L269 (2.76, 21.296) -> (2.76, 21.0285)
  line L270 (2.76, 21.0285) -> (2.7045, 21.0285)
  line L271 (2.7045, 21.0285) -> (2.7045, 19.7387)
  spline S301 degree 2 poles (2.7045, 19.7387) (2.7045, 19.6515) (2.7283, 19.6515) knots 0 0 0 1 1 1
  spline S302 degree 2 poles (2.7283, 19.6515) (2.7402, 19.6515) (2.76, 19.6693) knots 0 0 0 1 1 1
  line L272 (2.76, 19.6693) -> (2.76, 19.4078)
  spline S303 degree 2 poles (3.3267, 20.3727) (3.3267, 20.3073) (3.3267, 20.2657) knots 0 0 0 1 1 1
  line L273 (3.3267, 20.2657) -> (3.0592, 20.2657)
  spline S304 degree 2 poles (3.0592, 20.2657) (3.0592, 20.2419) (3.0592, 20.1963) knots 0 0 0 1 1 1
  spline S305 degree 2 poles (3.0592, 20.1963) (3.0592, 19.9764) (3.1206, 19.6416) (3.1622, 19.6416) knots 0 0 0 1 2 2 2
  spline S306 degree 2 poles (3.1622, 19.6416) (3.2336, 19.6416) (3.2593, 20.024) knots 0 0 0 1 1 1
  line L274 (3.2593, 20.024) -> (3.3187, 20.024)
  spline S307 degree 2 poles (3.3187, 20.024) (3.291, 19.39) (3.1682, 19.39) knots 0 0 0 1 1 1
  spline S308 degree 2 poles (3.1682, 19.39) (2.9978, 19.39) (2.9978, 20.3786) knots 0 0 0 1 1 1
  spline S309 degree 2 poles (2.9978, 20.3786) (2.9978, 20.8046) (3.0909, 21.3475) (3.1642, 21.3475) knots 0 0 0 1 2 2 2
  spline S310 degree 2 poles (3.1642, 21.3475) (3.2355, 21.3475) (3.2771, 21.1256) knots 0 0 0 1 1 1
  spline S311 degree 2 poles (3.2771, 21.1256) (3.3267, 20.87) (3.3267, 20.3727) knots 0 0 0 1 1 1
  spline S312 degree 2 poles (3.2653, 20.5233) (3.2534, 21.1097) (3.1662, 21.1097) knots 0 0 0 1 1 1
  spline S313 degree 2 poles (3.1662, 21.1097) (3.075, 21.1097) (3.0632, 20.5233) knots 0 0 0 1 1 1
  line L275 (3.0632, 20.5233) -> (3.2653, 20.5233)
  spline S314 degree 2 poles (3.7289, 19.4177) (3.7071, 19.388) (3.6833, 19.388) knots 0 0 0 1 1 1
  spline S315 degree 2 poles (3.6833, 19.388) (3.6655, 19.388) (3.6318, 19.5584) (3.6298, 19.6515) knots 0 0 0 1 2 2 2
  spline S316 degree 2 poles (3.6298, 19.6515) (3.5664, 19.388) (3.507, 19.388) knots 0 0 0 1 1 1
  spline S317 degree 2 poles (3.507, 19.388) (3.4515, 19.388) (3.3861, 19.6733) (3.3861, 19.9249) knots 0 0 0 1 2 2 2
  spline S318 degree 2 poles (3.3861, 19.9249) (3.3861, 20.3984) (3.499, 20.4757) knots 0 0 0 1 1 1
  line L276 (3.499, 20.4757) -> (3.6041, 20.5451)
  spline S319 degree 2 poles (3.6041, 20.5451) (3.6278, 20.5629) (3.6278, 20.7452) knots 0 0 0 1 1 1
  spline S320 degree 2 poles (3.6278, 20.7452) (3.6278, 20.8977) (3.6258, 20.9215) knots 0 0 0 1 1 1